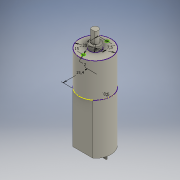
# Autodesk Inventor part: motor20
Saved by Autodesk Inventor 2020 (Build 240168000, 168)
## iProperties
Created: 2024-09-09
Part Number: motor20
Material: Типовые
Document SubType Name: Modeling
Designer: Ivan
Density: 1 g/cm^3
Appearance: Сталь — литейная
Mass: 15.2753 g
Surface Area: 41.6755 cm^2
Volume: 15.2753 cm^3
Author: Ivan
Autodesk Inventor part; units mm, degrees
ref_plane "YZ Plane" through (0, 0, 0) normal (1, 0, 0) x (0, 1, 0)
ref_plane "XZ Plane" through (0, 0, 0) normal (0, 1, 0) x (-1, 0, 0)
ref_plane "XY Plane" through (0, 0, 0) normal (0, 0, 1) x (1, 0, 0)
sketch "Эскиз1" plane through (0, 0, 0) normal (0, 1, 0) x (-1, 0, 0)
  circle A0 centre (0, 0) radius 10
  circle A1 centre (0, 0) radius 3.5
  circle A2 centre (0, 0) radius 2
  dimension "d0" = 20
  dimension "d1" = 7
  dimension "d2" = 4
  constraints: 3 centre point, 3 coincident
  measures "d0" diameter of A0
  measures "d1" diameter of A1
  measures "d2" diameter of A2
extrude "Выдавливание1" add sketch "Эскиз1" against normal blind 21.6 contours A0 | A1 | A2
extrude "Выдавливание2" add sketch "Эскиз1" along normal blind 3 contours A1
extrude "Выдавливание3" add sketch "Эскиз1" along normal blind 10.5 contours A2
sketch "Эскиз2" plane through (0, 10.5, 0) normal (0, 1, 0) x (1, 0, 0)
  circle A0 centre (0, 0) radius 2 projected
  circle A1 centre (0, 0) radius 2 projected
  circle A2 centre (0, 0) radius 3.5 projected
  line L0 (-3.1623, -1.5) -> (3.1623, -1.5)
  point P0 (0, 2)
  point P1 (0, 3.5)
  point P2 (1.3229, -1.5)
  point P3 (-1.3229, -1.5)
  dimension "d9" = 1.5
  constraints: 3 point on circle, 2 end point, 1 horizontal, 1 vertical alignment, 1 other
  measures "d9" distance from line of L0 point (0, 0)
extrude "Выдавливание4" cut sketch "Эскиз2" against normal blind 7 contours L0 A0 picked at (0.3089, -1.5908)
sketch "Эскиз3" plane through (0, -21.6, 0) normal (0, -1, 0) x (1, 0, 0)
  line L0 (6.3804, -7.7) -> (-6.3804, -7.7)
  line L1 (-6.3804, -7.7) -> (-6.3804, 7.7)
  line L2 (-6.3804, 7.7) -> (6.3804, 7.7)
  line L3 (6.3804, 7.7) -> (6.3804, -7.7)
  circle A0 centre (0, 0) radius 10 projected
  arc A1 (6.3804, -7.7) -> (6.3804, 7.7) centre (0, 0) ccw
  arc A2 (-6.3804, 7.7) -> (-6.3804, -7.7) centre (0, 0) ccw
  line L4 (5.3804, 0.25) -> (7.3804, 0.25)
  line L5 (7.3804, 0.25) -> (7.3804, -0.25)
  line L6 (7.3804, -0.25) -> (5.3804, -0.25)
  line L7 (5.3804, -0.25) -> (5.3804, 0.25)
  line L8 (5.3804, 0.25) -> (7.3804, -0.25) construction
  line L9 (0, -7.7) -> (0, 7.7) construction
  line L10 (-5.3804, 0.25) -> (-7.3804, 0.25)
  line L11 (-7.3804, 0.25) -> (-7.3804, -0.25)
  line L12 (-7.3804, -0.25) -> (-5.3804, -0.25)
  line L13 (-5.3804, -0.25) -> (-5.3804, 0.25)
  point P0 (6.3804, 0)
  point P1 (-6.3804, -7.7)
  dimension "d12" = 15.4
  dimension "d13" = 2
  dimension "d14" = 0.5
  constraints: 28 end point, 7 point on circle, 4 midpoint, 4 parallel, 4 symmetric about line, 2 centre point, 2 coincident, 2 horizontal, 2 perpendicular
  measures "d12" distance of L0.end L1.end
  measures "d13" distance of L5.end L6.end
  measures "d14" distance of L4.end L5.end
extrude "Выдавливание5" add sketch "Эскиз3" along normal blind 36 contours L6 L7 L4 L3 | L3 L4 L5 L6 | L12 L11 L10 L1 | L1 L10 L13 L12
extrude "Выдавливание6" add sketch "Эскиз3" along normal blind 32 contours L0 L1 L12 L13 L10 L2 L3 L4 L7 L6 | L3 L6 L5 L4 A0 | A0 L1 L10 L11 L12
sketch "Эскиз4" plane through (0, -53.6, 0) normal (0, -1, 0) x (1, 0, 0)
  circle A0 centre (0, 0) radius 2 projected
  circle A1 centre (0, 0) radius 3.1
  dimension "d19" = 6.2
  constraints: 1 centre point, 1 coincident
  measures "d19" diameter of A1
extrude "Выдавливание7" add sketch "Эскиз4" along normal blind 2.1 contours A0 | A1
sketch "Эскиз5" plane through (0, 0, 0) normal (0, 1, 0) x (1, 0, 0)
  circle A0 centre (0, 0) radius 10 construction
  line L0 (0, 10) -> (0, -10) construction
  circle A1 centre (0, 7.5) radius 1
  circle A2 centre (0, -7.5) radius 1
  dimension "d22" = 7.5
  dimension "d23" = 15
  dimension "d24" = 2
  constraints: 2 centre point, 2 end point, 2 point on circle, 2 point on line, 1 equal radius, 1 vertical
  measures "d22" distance of point (0, 0) A1.centre
  measures "d23" distance of A2.centre A1.centre
  measures "d24" diameter of A2
hole "Отверстие1" at (0, 0, 7.5) direction (0, -1, 0) diameter 2 depth 8 tip angle 118
hole "Отверстие2" at (0, 0, -7.5) direction (0, -1, 0) diameter 2 depth 8 tip angle 118
